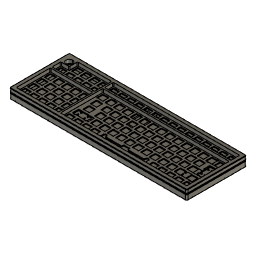
Varanidae (Autodesk Fusion 360 design; units mm, degrees)
Autodesk Fusion 360 part; units mm, degrees
(part 1 of 5)
sketch "スケッチ1" plane through (0, 0, 0) normal (0, 0, 1) x (1, 0, 0) in component "CasePlateDefault"
  spline S0 degree 3 poles (190.3558, 19.6941) (190.3558, 19.419) (190.1308, 19.194) (189.8555, 19.194) knots 0 0 0 0 1 1 1 1
  line L0 (189.8555, 19.194) -> (176.8555, 19.194)
  spline S1 degree 3 poles (176.8555, 19.194) (176.5806, 19.194) (176.3556, 19.419) (176.3556, 19.6941) knots 2 2 2 2 3 3 3 3
  line L1 (176.3556, 19.6941) -> (176.3556, 32.6938)
  spline S2 degree 3 poles (176.3556, 32.6938) (176.3556, 32.9689) (176.5806, 33.1939) (176.8555, 33.1939) knots 4 4 4 4 5 5 5 5
  line L2 (176.8555, 33.1939) -> (189.8555, 33.1939)
  spline S3 degree 3 poles (189.8555, 33.1939) (190.1308, 33.1939) (190.3558, 32.9689) (190.3558, 32.6938) knots 6 6 6 6 7 7 7 7
  line L3 (190.3558, 32.6938) -> (190.3558, 19.6941)
  spline S4 degree 3 poles (148.2805, 0.144) (148.0055, 0.144) (147.7806, 0.369) (147.7806, 0.6441) knots 0 0 0 0 1 1 1 1
  line L4 (147.7806, 0.6441) -> (147.7806, 13.6438)
  spline S5 degree 3 poles (147.7806, 13.6438) (147.7806, 13.9189) (148.0055, 14.1438) (148.2805, 14.1438) knots 2 2 2 2 3 3 3 3
  line L5 (148.2805, 14.1438) -> (161.2805, 14.1438)
  spline S6 degree 3 poles (161.2805, 14.1438) (161.5558, 14.1438) (161.7808, 13.9189) (161.7808, 13.6438) knots 4 4 4 4 5 5 5 5
  line L6 (161.7808, 13.6438) -> (161.7808, 0.6441)
  spline S7 degree 3 poles (161.7808, 0.6441) (161.7808, 0.369) (161.5558, 0.144) (161.2805, 0.144) knots 6 6 6 6 7 7 7 7
  line L7 (161.2805, 0.144) -> (148.2805, 0.144)
  spline S8 degree 3 poles (137.9686, -37.456) (137.9686, -37.7311) (137.7436, -37.956) (137.4684, -37.956) knots 0 0 0 0 1 1 1 1
  line L8 (137.4684, -37.956) -> (124.4686, -37.956)
  spline S9 degree 3 poles (124.4686, -37.956) (124.1937, -37.956) (123.9687, -37.7311) (123.9687, -37.456) knots 2 2 2 2 3 3 3 3
  line L9 (123.9687, -37.456) -> (123.9687, -24.4562)
  spline S10 degree 3 poles (123.9687, -24.4562) (123.9687, -24.1811) (124.1937, -23.9562) (124.4686, -23.9562) knots 4 4 4 4 5 5 5 5
  line L10 (124.4686, -23.9562) -> (137.4684, -23.9562)
  spline S11 degree 3 poles (137.4684, -23.9562) (137.7436, -23.9562) (137.9686, -24.1811) (137.9686, -24.4562) knots 6 6 6 6 7 7 7 7
  line L11 (137.9686, -24.4562) -> (137.9686, -37.456)
  spline S12 degree 3 poles (118.9186, -37.456) (118.9186, -37.7311) (118.6936, -37.956) (118.4183, -37.956) knots 0 0 0 0 1 1 1 1
  line L12 (118.4183, -37.956) -> (105.4186, -37.956)
  spline S13 degree 3 poles (105.4186, -37.956) (105.1437, -37.956) (104.9187, -37.7311) (104.9187, -37.456) knots 2 2 2 2 3 3 3 3
  line L13 (104.9187, -37.456) -> (104.9187, -24.4562)
  spline S14 degree 3 poles (104.9187, -24.4562) (104.9187, -24.1811) (105.1437, -23.9562) (105.4186, -23.9562) knots 4 4 4 4 5 5 5 5
  line L14 (105.4186, -23.9562) -> (118.4183, -23.9562)
  spline S15 degree 3 poles (118.4183, -23.9562) (118.6936, -23.9562) (118.9186, -24.1811) (118.9186, -24.4562) knots 6 6 6 6 7 7 7 7
  line L15 (118.9186, -24.4562) -> (118.9186, -37.456)
  spline S16 degree 3 poles (133.2057, -56.506) (133.2057, -56.7811) (132.9808, -57.006) (132.7055, -57.006) knots 0 0 0 0 1 1 1 1
  line L16 (132.7055, -57.006) -> (119.7054, -57.006)
  spline S17 degree 3 poles (119.7054, -57.006) (119.4305, -57.006) (119.2056, -56.7811) (119.2056, -56.506) knots 2 2 2 2 3 3 3 3
  line L17 (119.2056, -56.506) -> (119.2056, -43.5062)
  spline S18 degree 3 poles (119.2056, -43.5062) (119.2056, -43.2312) (119.4305, -43.0062) (119.7054, -43.0062) knots 4 4 4 4 5 5 5 5
  line L18 (119.7054, -43.0062) -> (132.7055, -43.0062)
  spline S19 degree 3 poles (132.7055, -43.0062) (132.9808, -43.0062) (133.2057, -43.2312) (133.2057, -43.5062) knots 6 6 6 6 7 7 7 7
  line L19 (133.2057, -43.5062) -> (133.2057, -56.506)
  line L20 (198.3818, 67.532) -> (-198.3818, 67.532)
  spline S20 degree 3 poles (-198.3818, 67.532) (-199.7568, 67.532) (-200.8816, 66.407) (-200.8816, 65.0321) knots 1 1 1 1 2 2 2 2
  line L21 (-200.8816, 65.0321) -> (-200.8816, -65.0319)
  spline S21 degree 3 poles (-200.8816, -65.0319) (-200.8816, -66.4072) (-199.7568, -67.532) (-198.3818, -67.532) knots 3 3 3 3 4 4 4 4
  line L22 (-198.3818, -67.532) -> (198.3818, -67.532)
  spline S22 degree 3 poles (198.3818, -67.532) (199.7564, -67.532) (200.8816, -66.4072) (200.8816, -65.0319) knots 5 5 5 5 6 6 6 6
  line L23 (200.8816, -65.0319) -> (200.8816, 65.0321)
  spline S23 degree 3 poles (200.8816, 65.0321) (200.8816, 66.407) (199.7564, 67.532) (198.3818, 67.532) knots 7 7 7 7 8 8 8 8
  spline S24 degree 3 poles (171.3058, -56.506) (171.3058, -56.7811) (171.0808, -57.006) (170.8055, -57.006) knots 0 0 0 0 1 1 1 1
  line L24 (170.8055, -57.006) -> (157.8055, -57.006)
  spline S25 degree 3 poles (157.8055, -57.006) (157.5305, -57.006) (157.3056, -56.7811) (157.3056, -56.506) knots 2 2 2 2 3 3 3 3
  line L25 (157.3056, -56.506) -> (157.3056, -43.5062)
  spline S26 degree 3 poles (157.3056, -43.5062) (157.3056, -43.2312) (157.5305, -43.0062) (157.8055, -43.0062) knots 4 4 4 4 5 5 5 5
  line L26 (157.8055, -43.0062) -> (170.8055, -43.0062)
  spline S27 degree 3 poles (170.8055, -43.0062) (171.0808, -43.0062) (171.3058, -43.2312) (171.3058, -43.5062) knots 6 6 6 6 7 7 7 7
  line L27 (171.3058, -43.5062) -> (171.3058, -56.506)
  spline S28 degree 3 poles (190.3558, -56.506) (190.3558, -56.7811) (190.1308, -57.006) (189.8555, -57.006) knots 0 0 0 0 1 1 1 1
  line L28 (189.8555, -57.006) -> (176.8555, -57.006)
  spline S29 degree 3 poles (176.8555, -57.006) (176.5806, -57.006) (176.3556, -56.7811) (176.3556, -56.506) knots 2 2 2 2 3 3 3 3
  line L29 (176.3556, -56.506) -> (176.3556, -43.5062)
  spline S30 degree 3 poles (176.3556, -43.5062) (176.3556, -43.2312) (176.5806, -43.0062) (176.8555, -43.0062) knots 4 4 4 4 5 5 5 5
  line L30 (176.8555, -43.0062) -> (189.8555, -43.0062)
  spline S31 degree 3 poles (189.8555, -43.0062) (190.1308, -43.0062) (190.3558, -43.2312) (190.3558, -43.5062) knots 6 6 6 6 7 7 7 7
  line L31 (190.3558, -43.5062) -> (190.3558, -56.506)
  spline S32 degree 3 poles (157.3056, 56.506) (157.3056, 56.7811) (157.5305, 57.006) (157.8055, 57.006) knots 0 0 0 0 1 1 1 1
  line L32 (157.8055, 57.006) -> (170.8055, 57.006)
  spline S33 degree 3 poles (170.8055, 57.006) (171.0808, 57.006) (171.3058, 56.7811) (171.3058, 56.506) knots 2 2 2 2 3 3 3 3
  line L33 (171.3058, 56.506) -> (171.3058, 43.5059)
  spline S34 degree 3 poles (171.3058, 43.5059) (171.3058, 43.2308) (171.0808, 43.0058) (170.8055, 43.0058) knots 4 4 4 4 5 5 5 5
  line L34 (170.8055, 43.0058) -> (157.8055, 43.0058)
  spline S35 degree 3 poles (157.8055, 43.0058) (157.5305, 43.0058) (157.3056, 43.2308) (157.3056, 43.5059) knots 6 6 6 6 7 7 7 7
  line L35 (157.3056, 43.5059) -> (157.3056, 56.506)
  spline S36 degree 3 poles (157.3056, 32.6938) (157.3056, 32.9689) (157.5305, 33.1939) (157.8055, 33.1939) knots 0 0 0 0 1 1 1 1
  line L36 (157.8055, 33.1939) -> (170.8055, 33.1939)
  spline S37 degree 3 poles (170.8055, 33.1939) (171.0808, 33.1939) (171.3058, 32.9689) (171.3058, 32.6938) knots 2 2 2 2 3 3 3 3
  line L37 (171.3058, 32.6938) -> (171.3058, 19.6941)
  spline S38 degree 3 poles (171.3058, 19.6941) (171.3058, 19.419) (171.0808, 19.194) (170.8055, 19.194) knots 4 4 4 4 5 5 5 5
  line L38 (170.8055, 19.194) -> (157.8055, 19.194)
  spline S39 degree 3 poles (157.8055, 19.194) (157.5305, 19.194) (157.3056, 19.419) (157.3056, 19.6941) knots 6 6 6 6 7 7 7 7
  line L39 (157.3056, 19.6941) -> (157.3056, 32.6938)
  spline S40 degree 3 poles (157.0186, -37.456) (157.0186, -37.7311) (156.7936, -37.956) (156.5184, -37.956) knots 0 0 0 0 1 1 1 1
  line L40 (156.5184, -37.956) -> (143.5186, -37.956)
  spline S41 degree 3 poles (143.5186, -37.956) (143.2437, -37.956) (143.0188, -37.7311) (143.0188, -37.456) knots 2 2 2 2 3 3 3 3
  line L41 (143.0188, -37.456) -> (143.0188, -24.4562)
  spline S42 degree 3 poles (143.0188, -24.4562) (143.0188, -24.1811) (143.2437, -23.9562) (143.5186, -23.9562) knots 4 4 4 4 5 5 5 5
  line L42 (143.5186, -23.9562) -> (156.5184, -23.9562)
  spline S43 degree 3 poles (156.5184, -23.9562) (156.7936, -23.9562) (157.0186, -24.1811) (157.0186, -24.4562) knots 6 6 6 6 7 7 7 7
  line L43 (157.0186, -24.4562) -> (157.0186, -37.456)
  line L44 (183.2117, -24.4562) -> (183.2117, -37.456)
  spline S44 degree 3 poles (183.2117, -37.456) (183.2117, -37.7311) (182.9867, -37.956) (182.7114, -37.956) knots 1 1 1 1 2 2 2 2
  line L45 (182.7114, -37.956) -> (169.7114, -37.956)
  spline S45 degree 3 poles (169.7114, -37.956) (169.4365, -37.956) (169.2115, -37.7311) (169.2115, -37.456) knots 3 3 3 3 4 4 4 4
  line L46 (169.2115, -37.456) -> (169.2115, -24.4562)
  spline S46 degree 3 poles (169.2115, -24.4562) (169.2115, -24.1811) (169.4365, -23.9562) (169.7114, -23.9562) knots 5 5 5 5 6 6 6 6
  line L47 (169.7114, -23.9562) -> (182.7114, -23.9562)
  spline S47 degree 3 poles (182.7114, -23.9562) (182.9867, -23.9562) (183.2117, -24.1811) (183.2117, -24.4562) knots 7 7 7 7 8 8 8 8
  spline S48 degree 3 poles (190.3558, 43.5059) (190.3558, 43.2308) (190.1308, 43.0058) (189.8555, 43.0058) knots 0 0 0 0 1 1 1 1
  line L48 (189.8555, 43.0058) -> (176.8555, 43.0058)
  spline S49 degree 3 poles (176.8555, 43.0058) (176.5806, 43.0058) (176.3556, 43.2308) (176.3556, 43.5059) knots 2 2 2 2 3 3 3 3
  line L49 (176.3556, 43.5059) -> (176.3556, 56.506)
  spline S50 degree 3 poles (176.3556, 56.506) (176.3556, 56.7811) (176.5806, 57.006) (176.8555, 57.006) knots 4 4 4 4 5 5 5 5
  line L50 (176.8555, 57.006) -> (189.8555, 57.006)
  spline S51 degree 3 poles (189.8555, 57.006) (190.1308, 57.006) (190.3558, 56.7811) (190.3558, 56.506) knots 6 6 6 6 7 7 7 7
  line L51 (190.3558, 56.506) -> (190.3558, 43.5059)
  spline S52 degree 3 poles (152.2558, -56.506) (152.2558, -56.7811) (152.0308, -57.006) (151.7555, -57.006) knots 0 0 0 0 1 1 1 1
  line L52 (151.7555, -57.006) -> (138.7554, -57.006)
  spline S53 degree 3 poles (138.7554, -57.006) (138.4805, -57.006) (138.2556, -56.7811) (138.2556, -56.506) knots 2 2 2 2 3 3 3 3
  line L53 (138.2556, -56.506) -> (138.2556, -43.5062)
  spline S54 degree 3 poles (138.2556, -43.5062) (138.2556, -43.2312) (138.4805, -43.0062) (138.7554, -43.0062) knots 4 4 4 4 5 5 5 5
  line L54 (138.7554, -43.0062) -> (151.7555, -43.0062)
  spline S55 degree 3 poles (151.7555, -43.0062) (152.0308, -43.0062) (152.2558, -43.2312) (152.2558, -43.5062) knots 6 6 6 6 7 7 7 7
  line L55 (152.2558, -43.5062) -> (152.2558, -56.506)
  spline S56 degree 3 poles (173.0045, -13.0311) (173.0045, -12.756) (173.2295, -12.531) (173.5044, -12.531) knots 0 0 0 0 1 1 1 1
  line L56 (173.5044, -12.531) -> (173.7042, -12.531)
  spline S57 degree 3 poles (173.7042, -12.531) (173.9795, -12.531) (174.2045, -12.3061) (174.2045, -12.031) knots 2 2 2 2 3 3 3 3
  line L57 (174.2045, -12.031) -> (174.2045, -11.3061)
  spline S58 degree 3 poles (174.2045, -11.3061) (174.2045, -11.031) (174.4294, -10.8061) (174.7044, -10.8061) knots 4 4 4 4 5 5 5 5
  line L58 (174.7044, -10.8061) -> (178.1746, -10.8061)
  spline S59 degree 3 poles (178.1746, -10.8061) (178.4499, -10.8061) (178.6748, -10.5811) (178.6748, -10.306) knots 6 6 6 6 7 7 7 7
  line L59 (178.6748, -10.306) -> (178.6748, -9.8811)
  spline S60 degree 3 poles (178.6748, -9.8811) (178.6748, -9.606) (178.4499, -9.381) (178.1746, -9.381) knots 8 8 8 8 9 9 9 9
  line L60 (178.1746, -9.381) -> (174.4746, -9.381)
  spline S61 degree 3 poles (174.4746, -9.381) (174.1996, -9.381) (173.9747, -9.156) (173.9747, -8.8809) knots 10 10 10 10 11 11 11 11
  line L61 (173.9747, -8.8809) -> (173.9747, 4.1188)
  spline S62 degree 3 poles (173.9747, 4.1188) (173.9747, 4.3939) (174.1996, 4.6188) (174.4746, 4.6188) knots 12 12 12 12 13 13 13 13
  line L62 (174.4746, 4.6188) -> (178.1746, 4.6188)
  spline S63 degree 3 poles (178.1746, 4.6188) (178.4499, 4.6188) (178.6748, 4.8438) (178.6748, 5.1189) knots 14 14 14 14 15 15 15 15
  line L63 (178.6748, 5.1189) -> (178.6748, 5.544)
  spline S64 degree 3 poles (178.6748, 5.544) (178.6748, 5.8191) (178.4499, 6.0441) (178.1746, 6.0441) knots 16 16 16 16 17 17 17 17
  line L64 (178.1746, 6.0441) -> (174.7044, 6.0441)
  spline S65 degree 3 poles (174.7044, 6.0441) (174.4294, 6.0441) (174.2045, 6.269) (174.2045, 6.5441) knots 18 18 18 18 19 19 19 19
  line L65 (174.2045, 6.5441) -> (174.2045, 7.269)
  spline S66 degree 3 poles (174.2045, 7.269) (174.2045, 7.5441) (173.9795, 7.769) (173.7042, 7.769) knots 20 20 20 20 21 21 21 21
  line L66 (173.7042, 7.769) -> (173.5044, 7.769)
  spline S67 degree 3 poles (173.5044, 7.769) (173.2295, 7.769) (173.0045, 7.994) (173.0045, 8.2691) knots 22 22 22 22 23 23 23 23
  line L67 (173.0045, 8.2691) -> (173.0045, 10.9189)
  spline S68 degree 3 poles (173.0045, 10.9189) (173.0045, 11.194) (173.2295, 11.4189) (173.5044, 11.4189) knots 24 24 24 24 25 25 25 25
  line L68 (173.5044, 11.4189) -> (173.7042, 11.4189)
  spline S69 degree 3 poles (173.7042, 11.4189) (173.9795, 11.4189) (174.2045, 11.6439) (174.2045, 11.919) knots 26 26 26 26 27 27 27 27
  line L69 (174.2045, 11.919) -> (174.2045, 12.644)
  spline S70 degree 3 poles (174.2045, 12.644) (174.2045, 12.9191) (174.4294, 13.1441) (174.7044, 13.1441) knots 28 28 28 28 29 29 29 29
  line L70 (174.7044, 13.1441) -> (179.9743, 13.1441)
  spline S71 degree 3 poles (179.9743, 13.1441) (180.2496, 13.1441) (180.4745, 13.2734) (180.4745, 13.5897) (180.6995, 13.7191) (180.9744, 13.7191) knots 30 30 30 30 31 31 32 32 32 32
  line L71 (180.9744, 13.7191) -> (182.7745, 13.7191)
  spline S72 degree 3 poles (182.7745, 13.7191) (183.0498, 13.7191) (183.2747, 13.5897) (183.2747, 13.2734) (183.4997, 13.1441) (183.7746, 13.1441) knots 33 33 33 33 34 34 35 35 35 35
  line L72 (183.7746, 13.1441) -> (186.5038, 13.1441)
  spline S73 degree 3 poles (186.5038, 13.1441) (186.7791, 13.1441) (187.004, 12.9191) (187.004, 12.644) knots 36 36 36 36 37 37 37 37
  line L73 (187.004, 12.644) -> (187.004, 6.5441)
  spline S74 degree 3 poles (187.004, 6.5441) (187.004, 6.269) (186.7791, 6.0441) (186.5038, 6.0441) knots 38 38 38 38 39 39 39 39
  line L74 (186.5038, 6.0441) -> (183.7746, 6.0441)
  spline S75 degree 3 poles (183.7746, 6.0441) (183.4997, 6.0441) (183.2747, 5.8191) (183.2747, 5.544) knots 40 40 40 40 41 41 41 41
  line L75 (183.2747, 5.544) -> (183.2747, 5.1189)
  spline S76 degree 3 poles (183.2747, 5.1189) (183.2747, 4.8438) (183.4997, 4.6188) (183.7746, 4.6188) knots 42 42 42 42 43 43 43 43
  line L76 (183.7746, 4.6188) -> (187.4743, 4.6188)
  spline S77 degree 3 poles (187.4743, 4.6188) (187.7496, 4.6188) (187.9745, 4.3939) (187.9745, 4.1188) knots 44 44 44 44 45 45 45 45
  line L77 (187.9745, 4.1188) -> (187.9745, -8.8809)
  spline S78 degree 3 poles (187.9745, -8.8809) (187.9745, -9.156) (187.7496, -9.381) (187.4743, -9.381) knots 46 46 46 46 47 47 47 47
  line L78 (187.4743, -9.381) -> (183.7746, -9.381)
  spline S79 degree 3 poles (183.7746, -9.381) (183.4997, -9.381) (183.2747, -9.606) (183.2747, -9.8811) knots 48 48 48 48 49 49 49 49
  line L79 (183.2747, -9.8811) -> (183.2747, -10.306)
  spline S80 degree 3 poles (183.2747, -10.306) (183.2747, -10.5811) (183.4997, -10.8061) (183.7746, -10.8061) knots 50 50 50 50 51 51 51 51
  line L80 (183.7746, -10.8061) -> (186.5038, -10.8061)
  spline S81 degree 3 poles (186.5038, -10.8061) (186.7791, -10.8061) (187.004, -11.031) (187.004, -11.3061) knots 52 52 52 52 53 53 53 53
  line L81 (187.004, -11.3061) -> (187.004, -17.406)
  spline S82 degree 3 poles (187.004, -17.406) (187.004, -17.6811) (186.7791, -17.9061) (186.5038, -17.9061) knots 54 54 54 54 55 55 55 55
  line L82 (186.5038, -17.9061) -> (183.7746, -17.9061)
  spline S83 degree 3 poles (183.7746, -17.9061) (183.4997, -17.9061) (183.2747, -18.0354) (183.2747, -18.1936) (183.2747, -18.3519) (183.0498, -18.4812) (182.7745, -18.4812) knots 56 56 56 56 57 57 57 58 58 58 58
  line L83 (182.7745, -18.4812) -> (180.9744, -18.4812)
  spline S84 degree 3 poles (180.9744, -18.4812) (180.6995, -18.4812) (180.4745, -18.3519) (180.4745, -18.1936) (180.4745, -18.0354) (180.2496, -17.9061) (179.9743, -17.9061) knots 59 59 59 59 60 60 60 61 61 61 61
  line L84 (179.9743, -17.9061) -> (174.7044, -17.9061)
  spline S85 degree 3 poles (174.7044, -17.9061) (174.4294, -17.9061) (174.2045, -17.6811) (174.2045, -17.406) knots 62 62 62 62 63 63 63 63
  line L85 (174.2045, -17.406) -> (174.2045, -16.681)
  spline S86 degree 3 poles (174.2045, -16.681) (174.2045, -16.4059) (173.9795, -16.1809) (173.7042, -16.1809) knots 64 64 64 64 65 65 65 65
  line L86 (173.7042, -16.1809) -> (173.5044, -16.1809)
  spline S87 degree 3 poles (173.5044, -16.1809) (173.2295, -16.1809) (173.0045, -15.956) (173.0045, -15.6809) knots 66 66 66 66 67 67 67 67
  line L87 (173.0045, -15.6809) -> (173.0045, -13.0311)
  spline S88 degree 3 poles (152.5438, -5.4062) (152.5438, -5.1311) (152.7687, -4.9062) (153.0436, -4.9062) knots 0 0 0 0 1 1 1 1
  line L88 (153.0436, -4.9062) -> (166.0434, -4.9062)
  spline S89 degree 3 poles (166.0434, -4.9062) (166.3186, -4.9062) (166.5436, -5.1311) (166.5436, -5.4062) knots 2 2 2 2 3 3 3 3
  line L89 (166.5436, -5.4062) -> (166.5436, -18.406)
  spline S90 degree 3 poles (166.5436, -18.406) (166.5436, -18.681) (166.3186, -18.906) (166.0434, -18.906) knots 4 4 4 4 5 5 5 5
  line L90 (166.0434, -18.906) -> (153.0436, -18.906)
  spline S91 degree 3 poles (153.0436, -18.906) (152.7687, -18.906) (152.5438, -18.681) (152.5438, -18.406) knots 6 6 6 6 7 7 7 7
  line L91 (152.5438, -18.406) -> (152.5438, -5.4062)
  spline S92 degree 3 poles (138.2556, 32.6938) (138.2556, 32.9689) (138.4805, 33.1939) (138.7554, 33.1939) knots 0 0 0 0 1 1 1 1
  line L92 (138.7554, 33.1939) -> (151.7555, 33.1939)
  spline S93 degree 3 poles (151.7555, 33.1939) (152.0308, 33.1939) (152.2558, 32.9689) (152.2558, 32.6938) knots 2 2 2 2 3 3 3 3
  line L93 (152.2558, 32.6938) -> (152.2558, 19.6941)
  spline S94 degree 3 poles (152.2558, 19.6941) (152.2558, 19.419) (152.0308, 19.194) (151.7555, 19.194) knots 4 4 4 4 5 5 5 5
  line L94 (151.7555, 19.194) -> (138.7554, 19.194)
  spline S95 degree 3 poles (138.7554, 19.194) (138.4805, 19.194) (138.2556, 19.419) (138.2556, 19.6941) knots 6 6 6 6 7 7 7 7
  line L95 (138.2556, 19.6941) -> (138.2556, 32.6938)
  spline S96 degree 3 poles (138.2556, 56.506) (138.2556, 56.7811) (138.4805, 57.006) (138.7554, 57.006) knots 0 0 0 0 1 1 1 1
  line L96 (138.7554, 57.006) -> (151.7555, 57.006)
  spline S97 degree 3 poles (151.7555, 57.006) (152.0308, 57.006) (152.2558, 56.7811) (152.2558, 56.506) knots 2 2 2 2 3 3 3 3
  line L97 (152.2558, 56.506) -> (152.2558, 43.5059)
  spline S98 degree 3 poles (152.2558, 43.5059) (152.2558, 43.2308) (152.0308, 43.0058) (151.7555, 43.0058) knots 4 4 4 4 5 5 5 5
  line L98 (151.7555, 43.0058) -> (138.7554, 43.0058)
  spline S99 degree 3 poles (138.7554, 43.0058) (138.4805, 43.0058) (138.2556, 43.2308) (138.2556, 43.5059) knots 6 6 6 6 7 7 7 7
  line L99 (138.2556, 43.5059) -> (138.2556, 56.506)
  spline S100 degree 3 poles (-71.2946, 32.6938) (-71.2946, 32.9689) (-71.0696, 33.1939) (-70.7947, 33.1939) knots 0 0 0 0 1 1 1 1
  line L100 (-70.7947, 33.1939) -> (-57.795, 33.1939)
  spline S101 degree 3 poles (-57.795, 33.1939) (-57.5197, 33.1939) (-57.2947, 32.9689) (-57.2947, 32.6938) knots 2 2 2 2 3 3 3 3
  line L101 (-57.2947, 32.6938) -> (-57.2947, 19.6941)
  spline S102 degree 3 poles (-57.2947, 19.6941) (-57.2947, 19.419) (-57.5197, 19.194) (-57.795, 19.194) knots 4 4 4 4 5 5 5 5
  line L102 (-57.795, 19.194) -> (-70.7947, 19.194)
  spline S103 degree 3 poles (-70.7947, 19.194) (-71.0696, 19.194) (-71.2946, 19.419) (-71.2946, 19.6941) knots 6 6 6 6 7 7 7 7
  line L103 (-71.2946, 19.6941) -> (-71.2946, 32.6938)
  spline S104 degree 3 poles (-71.2946, 56.506) (-71.2946, 56.7811) (-71.0696, 57.006) (-70.7947, 57.006) knots 0 0 0 0 1 1 1 1
  line L104 (-70.7947, 57.006) -> (-57.795, 57.006)
  spline S105 degree 3 poles (-57.795, 57.006) (-57.5197, 57.006) (-57.2947, 56.7811) (-57.2947, 56.506) knots 2 2 2 2 3 3 3 3
  line L105 (-57.2947, 56.506) -> (-57.2947, 43.5059)
  spline S106 degree 3 poles (-57.2947, 43.5059) (-57.2947, 43.2308) (-57.5197, 43.0058) (-57.795, 43.0058) knots 4 4 4 4 5 5 5 5
  line L106 (-57.795, 43.0058) -> (-70.7947, 43.0058)
  spline S107 degree 3 poles (-70.7947, 43.0058) (-71.0696, 43.0058) (-71.2946, 43.2308) (-71.2946, 43.5059) knots 6 6 6 6 7 7 7 7
  line L107 (-71.2946, 43.5059) -> (-71.2946, 56.506)
  line L108 (-69.2006, -5.4062) -> (-69.2006, -18.406)
  spline S108 degree 3 poles (-69.2006, -18.406) (-69.2006, -18.681) (-69.4256, -18.906) (-69.7009, -18.906) knots 1 1 1 1 2 2 2 2
  line L109 (-69.7009, -18.906) -> (-82.7006, -18.906)
  spline S109 degree 3 poles (-82.7006, -18.906) (-82.9755, -18.906) (-83.2005, -18.681) (-83.2005, -18.406) knots 3 3 3 3 4 4 4 4
  line L110 (-83.2005, -18.406) -> (-83.2005, -5.4062)
  spline S110 degree 3 poles (-83.2005, -5.4062) (-83.2005, -5.1311) (-82.9755, -4.9062) (-82.7006, -4.9062) knots 5 5 5 5 6 6 6 6
  line L111 (-82.7006, -4.9062) -> (-69.7009, -4.9062)
  spline S111 degree 3 poles (-69.7009, -4.9062) (-69.4256, -4.9062) (-69.2006, -5.1311) (-69.2006, -5.4062) knots 7 7 7 7 8 8 8 8
  line L112 (14.4305, 0.6441) -> (14.4305, 13.6438)
  spline S112 degree 3 poles (14.4305, 13.6438) (14.4305, 13.9189) (14.6554, 14.1438) (14.9304, 14.1438) knots 1 1 1 1 2 2 2 2
  line L113 (14.9304, 14.1438) -> (27.9304, 14.1438)
  spline S113 degree 3 poles (27.9304, 14.1438) (28.2057, 14.1438) (28.4307, 13.9189) (28.4307, 13.6438) knots 3 3 3 3 4 4 4 4
  line L114 (28.4307, 13.6438) -> (28.4307, 0.6441)
  spline S114 degree 3 poles (28.4307, 0.6441) (28.4307, 0.369) (28.2057, 0.144) (27.9304, 0.144) knots 5 5 5 5 6 6 6 6
  line L115 (27.9304, 0.144) -> (14.9304, 0.144)
  spline S115 degree 3 poles (14.9304, 0.144) (14.6554, 0.144) (14.4305, 0.369) (14.4305, 0.6441) knots 7 7 7 7 8 8 8 8
  spline S116 degree 3 poles (133.4937, -5.4062) (133.4937, -5.1311) (133.7187, -4.9062) (133.9936, -4.9062) knots 0 0 0 0 1 1 1 1
  line L116 (133.9936, -4.9062) -> (146.9934, -4.9062)
  spline S117 degree 3 poles (146.9934, -4.9062) (147.2686, -4.9062) (147.4936, -5.1311) (147.4936, -5.4062) knots 2 2 2 2 3 3 3 3
  line L117 (147.4936, -5.4062) -> (147.4936, -18.406)
  spline S118 degree 3 poles (147.4936, -18.406) (147.4936, -18.681) (147.2686, -18.906) (146.9934, -18.906) knots 4 4 4 4 5 5 5 5
  line L118 (146.9934, -18.906) -> (133.9936, -18.906)
  spline S119 degree 3 poles (133.9936, -18.906) (133.7187, -18.906) (133.4937, -18.681) (133.4937, -18.406) knots 6 6 6 6 7 7 7 7
  line L119 (133.4937, -18.406) -> (133.4937, -5.4062)
  line L120 (-71.5816, 13.6438) -> (-71.5816, 0.6441)
  spline S120 degree 3 poles (-71.5816, 0.6441) (-71.5816, 0.369) (-71.8065, 0.144) (-72.0818, 0.144) knots 1 1 1 1 2 2 2 2
  line L121 (-72.0818, 0.144) -> (-85.0819, 0.144)
  spline S121 degree 3 poles (-85.0819, 0.144) (-85.3568, 0.144) (-85.5817, 0.369) (-85.5817, 0.6441) knots 3 3 3 3 4 4 4 4
  line L122 (-85.5817, 0.6441) -> (-85.5817, 13.6438)
  spline S122 degree 3 poles (-85.5817, 13.6438) (-85.5817, 13.9189) (-85.3568, 14.1438) (-85.0819, 14.1438) knots 5 5 5 5 6 6 6 6
  line L123 (-85.0819, 14.1438) -> (-72.0818, 14.1438)
  spline S123 degree 3 poles (-72.0818, 14.1438) (-71.8065, 14.1438) (-71.5816, 13.9189) (-71.5816, 13.6438) knots 7 7 7 7 8 8 8 8
  spline S124 degree 3 poles (47.7687, -24.4562) (47.7687, -24.1811) (47.9937, -23.9562) (48.2686, -23.9562) knots 0 0 0 0 1 1 1 1
  line L124 (48.2686, -23.9562) -> (61.2673, -23.9562)
  spline S125 degree 3 poles (61.2673, -23.9562) (61.5425, -23.9562) (61.7675, -24.1811) (61.7675, -24.4562) knots 2 2 2 2 3 3 3 3
  line L125 (61.7675, -24.4562) -> (61.7675, -37.456)
  spline S126 degree 3 poles (61.7675, -37.456) (61.7675, -37.7311) (61.5425, -37.956) (61.2673, -37.956) knots 4 4 4 4 5 5 5 5
  line L126 (61.2673, -37.956) -> (48.2686, -37.956)
  spline S127 degree 3 poles (48.2686, -37.956) (47.9937, -37.956) (47.7687, -37.7311) (47.7687, -37.456) knots 6 6 6 6 7 7 7 7
  line L127 (47.7687, -37.456) -> (47.7687, -24.4562)
  spline S128 degree 3 poles (-90.3446, 56.506) (-90.3446, 56.7811) (-90.1196, 57.006) (-89.8447, 57.006) knots 0 0 0 0 1 1 1 1
  line L128 (-89.8447, 57.006) -> (-76.845, 57.006)
  spline S129 degree 3 poles (-76.845, 57.006) (-76.5697, 57.006) (-76.3447, 56.7811) (-76.3447, 56.506) knots 2 2 2 2 3 3 3 3
  line L129 (-76.3447, 56.506) -> (-76.3447, 43.5059)
  spline S130 degree 3 poles (-76.3447, 43.5059) (-76.3447, 43.2308) (-76.5697, 43.0058) (-76.845, 43.0058) knots 4 4 4 4 5 5 5 5
  line L130 (-76.845, 43.0058) -> (-89.8447, 43.0058)
  spline S131 degree 3 poles (-89.8447, 43.0058) (-90.1196, 43.0058) (-90.3446, 43.2308) (-90.3446, 43.5059) knots 6 6 6 6 7 7 7 7
  line L131 (-90.3446, 43.5059) -> (-90.3446, 56.506)
  spline S132 degree 3 poles (119.2056, 56.506) (119.2056, 56.7811) (119.4305, 57.006) (119.7054, 57.006) knots 0 0 0 0 1 1 1 1
  line L132 (119.7054, 57.006) -> (132.7055, 57.006)
  spline S133 degree 3 poles (132.7055, 57.006) (132.9808, 57.006) (133.2057, 56.7811) (133.2057, 56.506) knots 2 2 2 2 3 3 3 3
  line L133 (133.2057, 56.506) -> (133.2057, 43.5059)
  spline S134 degree 3 poles (133.2057, 43.5059) (133.2057, 43.2308) (132.9808, 43.0058) (132.7055, 43.0058) knots 4 4 4 4 5 5 5 5
  line L134 (132.7055, 43.0058) -> (119.7054, 43.0058)
  spline S135 degree 3 poles (119.7054, 43.0058) (119.4305, 43.0058) (119.2056, 43.2308) (119.2056, 43.5059) knots 6 6 6 6 7 7 7 7
  line L135 (119.2056, 43.5059) -> (119.2056, 56.506)
  spline S136 degree 3 poles (-18.9064, -5.4062) (-18.9064, -5.1311) (-18.6814, -4.9062) (-18.4065, -4.9062) knots 0 0 0 0 1 1 1 1
  line L136 (-18.4065, -4.9062) -> (-5.4067, -4.9062)
  spline S137 degree 3 poles (-5.4067, -4.9062) (-5.1315, -4.9062) (-4.9065, -5.1311) (-4.9065, -5.4062) knots 2 2 2 2 3 3 3 3
  line L137 (-4.9065, -5.4062) -> (-4.9065, -18.406)
  spline S138 degree 3 poles (-4.9065, -18.406) (-4.9065, -18.681) (-5.1315, -18.906) (-5.4067, -18.906) knots 4 4 4 4 5 5 5 5
  line L138 (-5.4067, -18.906) -> (-18.4065, -18.906)
  spline S139 degree 3 poles (-18.4065, -18.906) (-18.6814, -18.906) (-18.9064, -18.681) (-18.9064, -18.406) knots 6 6 6 6 7 7 7 7
  line L139 (-18.9064, -18.406) -> (-18.9064, -5.4062)
  spline S140 degree 3 poles (28.7187, -24.4562) (28.7187, -24.1811) (28.9436, -23.9562) (29.2186, -23.9562) knots 0 0 0 0 1 1 1 1
  line L140 (29.2186, -23.9562) -> (42.2183, -23.9562)
  spline S141 degree 3 poles (42.2183, -23.9562) (42.4936, -23.9562) (42.7185, -24.1811) (42.7185, -24.4562) knots 2 2 2 2 3 3 3 3
  line L141 (42.7185, -24.4562) -> (42.7185, -37.456)
  spline S142 degree 3 poles (42.7185, -37.456) (42.7185, -37.7311) (42.4936, -37.956) (42.2183, -37.956) knots 4 4 4 4 5 5 5 5
  line L142 (42.2183, -37.956) -> (29.2186, -37.956)
  spline S143 degree 3 poles (29.2186, -37.956) (28.9436, -37.956) (28.7187, -37.7311) (28.7187, -37.456) knots 6 6 6 6 7 7 7 7
  line L143 (28.7187, -37.456) -> (28.7187, -24.4562)
  spline S144 degree 3 poles (-176.3566, -56.506) (-176.3566, -56.7811) (-176.5816, -57.006) (-176.8568, -57.006) knots 0 0 0 0 1 1 1 1
  line L144 (-176.8568, -57.006) -> (-189.8569, -57.006)
  spline S145 degree 3 poles (-189.8569, -57.006) (-190.1318, -57.006) (-190.3568, -56.7811) (-190.3568, -56.506) knots 2 2 2 2 3 3 3 3
  line L145 (-190.3568, -56.506) -> (-190.3568, -43.5062)
  spline S146 degree 3 poles (-190.3568, -43.5062) (-190.3568, -43.2312) (-190.1318, -43.0062) (-189.8569, -43.0062) knots 4 4 4 4 5 5 5 5
  line L146 (-189.8569, -43.0062) -> (-176.8568, -43.0062)
  spline S147 degree 3 poles (-176.8568, -43.0062) (-176.5816, -43.0062) (-176.3566, -43.2312) (-176.3566, -43.5062) knots 6 6 6 6 7 7 7 7
  line L147 (-176.3566, -43.5062) -> (-176.3566, -56.506)
  line L148 (52.5305, 0.6441) -> (52.5305, 13.6438)
  spline S148 degree 3 poles (52.5305, 13.6438) (52.5305, 13.9189) (52.7555, 14.1438) (53.0304, 14.1438) knots 1 1 1 1 2 2 2 2
  line L149 (53.0304, 14.1438) -> (66.0305, 14.1438)
  spline S149 degree 3 poles (66.0305, 14.1438) (66.3057, 14.1438) (66.5307, 13.9189) (66.5307, 13.6438) knots 3 3 3 3 4 4 4 4
  line L150 (66.5307, 13.6438) -> (66.5307, 0.6441)
  spline S150 degree 3 poles (66.5307, 0.6441) (66.5307, 0.369) (66.3057, 0.144) (66.0305, 0.144) knots 5 5 5 5 6 6 6 6
  line L151 (66.0305, 0.144) -> (53.0304, 0.144)
  spline S151 degree 3 poles (53.0304, 0.144) (52.7555, 0.144) (52.5305, 0.369) (52.5305, 0.6441) knots 7 7 7 7 8 8 8 8
  line L152 (-4.6195, 0.6441) -> (-4.6195, 13.6438)
  spline S152 degree 3 poles (-4.6195, 13.6438) (-4.6195, 13.9189) (-4.3946, 14.1438) (-4.1196, 14.1438) knots 1 1 1 1 2 2 2 2
  line L153 (-4.1196, 14.1438) -> (8.8804, 14.1438)
  spline S153 degree 3 poles (8.8804, 14.1438) (9.1557, 14.1438) (9.3807, 13.9189) (9.3807, 13.6438) knots 3 3 3 3 4 4 4 4
  line L154 (9.3807, 13.6438) -> (9.3807, 0.6441)
  spline S154 degree 3 poles (9.3807, 0.6441) (9.3807, 0.369) (9.1557, 0.144) (8.8804, 0.144) knots 5 5 5 5 6 6 6 6
  line L155 (8.8804, 0.144) -> (-4.1196, 0.144)
  spline S155 degree 3 poles (-4.1196, 0.144) (-4.3946, 0.144) (-4.6195, 0.369) (-4.6195, 0.6441) knots 7 7 7 7 8 8 8 8
  spline S156 degree 3 poles (-176.3566, -37.456) (-176.3566, -37.7311) (-176.5816, -37.956) (-176.8568, -37.956) knots 0 0 0 0 1 1 1 1
  line L156 (-176.8568, -37.956) -> (-189.8569, -37.956)
  spline S157 degree 3 poles (-189.8569, -37.956) (-190.1318, -37.956) (-190.3568, -37.7311) (-190.3568, -37.456) knots 2 2 2 2 3 3 3 3
  line L157 (-190.3568, -37.456) -> (-190.3568, -24.4562)
  spline S158 degree 3 poles (-190.3568, -24.4562) (-190.3568, -24.1811) (-190.1318, -23.9562) (-189.8569, -23.9562) knots 4 4 4 4 5 5 5 5
  line L158 (-189.8569, -23.9562) -> (-176.8568, -23.9562)
  spline S159 degree 3 poles (-176.8568, -23.9562) (-176.5816, -23.9562) (-176.3566, -24.1811) (-176.3566, -24.4562) knots 6 6 6 6 7 7 7 7
  line L159 (-176.3566, -24.4562) -> (-176.3566, -37.456)
  spline S160 degree 3 poles (-176.3566, -18.406) (-176.3566, -18.681) (-176.5816, -18.906) (-176.8568, -18.906) knots 0 0 0 0 1 1 1 1
  line L160 (-176.8568, -18.906) -> (-189.8569, -18.906)
  spline S161 degree 3 poles (-189.8569, -18.906) (-190.1318, -18.906) (-190.3568, -18.681) (-190.3568, -18.406) knots 2 2 2 2 3 3 3 3
  line L161 (-190.3568, -18.406) -> (-190.3568, -5.4062)
  spline S162 degree 3 poles (-190.3568, -5.4062) (-190.3568, -5.1311) (-190.1318, -4.9062) (-189.8569, -4.9062) knots 4 4 4 4 5 5 5 5
  line L162 (-189.8569, -4.9062) -> (-176.8568, -4.9062)
  spline S163 degree 3 poles (-176.8568, -4.9062) (-176.5816, -4.9062) (-176.3566, -5.1311) (-176.3566, -5.4062) knots 6 6 6 6 7 7 7 7
  line L163 (-176.3566, -5.4062) -> (-176.3566, -18.406)
  spline S164 degree 3 poles (-176.3566, 24.4559) (-176.3566, 24.1808) (-176.5816, 23.9558) (-176.8568, 23.9558) knots 0 0 0 0 1 1 1 1
  line L164 (-176.8568, 23.9558) -> (-189.8569, 23.9558)
  spline S165 degree 3 poles (-189.8569, 23.9558) (-190.1318, 23.9558) (-190.3568, 24.1808) (-190.3568, 24.4559) knots 2 2 2 2 3 3 3 3
  line L165 (-190.3568, 24.4559) -> (-190.3568, 37.456)
  spline S166 degree 3 poles (-190.3568, 37.456) (-190.3568, 37.7311) (-190.1318, 37.956) (-189.8569, 37.956) knots 4 4 4 4 5 5 5 5
  line L166 (-189.8569, 37.956) -> (-176.8568, 37.956)
  spline S167 degree 3 poles (-176.8568, 37.956) (-176.5816, 37.956) (-176.3566, 37.7311) (-176.3566, 37.456) knots 6 6 6 6 7 7 7 7
  line L167 (-176.3566, 37.456) -> (-176.3566, 24.4559)
  spline S168 degree 3 poles (-9.3813, -24.4562) (-9.3813, -24.1811) (-9.1564, -23.9562) (-8.8815, -23.9562) knots 0 0 0 0 1 1 1 1
  line L168 (-8.8815, -23.9562) -> (4.1183, -23.9562)
  spline S169 degree 3 poles (4.1183, -23.9562) (4.3935, -23.9562) (4.6185, -24.1811) (4.6185, -24.4562) knots 2 2 2 2 3 3 3 3
  line L169 (4.6185, -24.4562) -> (4.6185, -37.456)
  spline S170 degree 3 poles (4.6185, -37.456) (4.6185, -37.7311) (4.3935, -37.956) (4.1183, -37.956) knots 4 4 4 4 5 5 5 5
  line L170 (4.1183, -37.956) -> (-8.8815, -37.956)
  spline S171 degree 3 poles (-8.8815, -37.956) (-9.1564, -37.956) (-9.3813, -37.7311) (-9.3813, -37.456) knots 6 6 6 6 7 7 7 7
  line L171 (-9.3813, -37.456) -> (-9.3813, -24.4562)
  spline S172 degree 3 poles (-14.1445, 32.6938) (-14.1445, 32.9689) (-13.9196, 33.1939) (-13.6447, 33.1939) knots 0 0 0 0 1 1 1 1
  line L172 (-13.6447, 33.1939) -> (-0.6446, 33.1939)
  spline S173 degree 3 poles (-0.6446, 33.1939) (-0.3693, 33.1939) (-0.1443, 32.9689) (-0.1443, 32.6938) knots 2 2 2 2 3 3 3 3
  line L173 (-0.1443, 32.6938) -> (-0.1443, 19.6941)
  spline S174 degree 3 poles (-0.1443, 19.6941) (-0.1443, 19.419) (-0.3693, 19.194) (-0.6446, 19.194) knots 4 4 4 4 5 5 5 5
  line L174 (-0.6446, 19.194) -> (-13.6447, 19.194)
  spline S175 degree 3 poles (-13.6447, 19.194) (-13.9196, 19.194) (-14.1445, 19.419) (-14.1445, 19.6941) knots 6 6 6 6 7 7 7 7
  line L175 (-14.1445, 19.6941) -> (-14.1445, 32.6938)
  spline S176 degree 3 poles (-176.3566, 0.6441) (-176.3566, 0.369) (-176.5816, 0.144) (-176.8568, 0.144) knots 0 0 0 0 1 1 1 1
  line L176 (-176.8568, 0.144) -> (-189.8569, 0.144)
  spline S177 degree 3 poles (-189.8569, 0.144) (-190.1318, 0.144) (-190.3568, 0.369) (-190.3568, 0.6441) knots 2 2 2 2 3 3 3 3
  line L177 (-190.3568, 0.6441) -> (-190.3568, 13.6438)
  spline S178 degree 3 poles (-190.3568, 13.6438) (-190.3568, 13.9189) (-190.1318, 14.1438) (-189.8569, 14.1438) knots 4 4 4 4 5 5 5 5
  line L178 (-189.8569, 14.1438) -> (-176.8568, 14.1438)
  spline S179 degree 3 poles (-176.8568, 14.1438) (-176.5816, 14.1438) (-176.3566, 13.9189) (-176.3566, 13.6438) knots 6 6 6 6 7 7 7 7
  line L179 (-176.3566, 13.6438) -> (-176.3566, 0.6441)
  spline S180 degree 3 poles (-157.3066, -56.506) (-157.3066, -56.7811) (-157.5316, -57.006) (-157.8068, -57.006) knots 0 0 0 0 1 1 1 1
  line L180 (-157.8068, -57.006) -> (-170.8069, -57.006)
  spline S181 degree 3 poles (-170.8069, -57.006) (-171.0818, -57.006) (-171.3068, -56.7811) (-171.3068, -56.506) knots 2 2 2 2 3 3 3 3
  line L181 (-171.3068, -56.506) -> (-171.3068, -43.5062)
  spline S182 degree 3 poles (-171.3068, -43.5062) (-171.3068, -43.2312) (-171.0818, -43.0062) (-170.8069, -43.0062) knots 4 4 4 4 5 5 5 5
  line L182 (-170.8069, -43.0062) -> (-157.8068, -43.0062)
  spline S183 degree 3 poles (-157.8068, -43.0062) (-157.5316, -43.0062) (-157.3066, -43.2312) (-157.3066, -43.5062) knots 6 6 6 6 7 7 7 7
  line L183 (-157.3066, -43.5062) -> (-157.3066, -56.506)
  spline S184 degree 3 poles (62.0555, 56.506) (62.0555, 56.7811) (62.2805, 57.006) (62.5554, 57.006) knots 0 0 0 0 1 1 1 1
  line L184 (62.5554, 57.006) -> (75.5555, 57.006)
  spline S185 degree 3 poles (75.5555, 57.006) (75.8307, 57.006) (76.0557, 56.7811) (76.0557, 56.506) knots 2 2 2 2 3 3 3 3
  line L185 (76.0557, 56.506) -> (76.0557, 43.5059)
  spline S186 degree 3 poles (76.0557, 43.5059) (76.0557, 43.2308) (75.8307, 43.0058) (75.5555, 43.0058) knots 4 4 4 4 5 5 5 5
  line L186 (75.5555, 43.0058) -> (62.5554, 43.0058)
  spline S187 degree 3 poles (62.5554, 43.0058) (62.2805, 43.0058) (62.0555, 43.2308) (62.0555, 43.5059) knots 6 6 6 6 7 7 7 7
  line L187 (62.0555, 43.5059) -> (62.0555, 56.506)
  line L188 (33.4805, 0.6441) -> (33.4805, 13.6438)
  spline S188 degree 3 poles (33.4805, 13.6438) (33.4805, 13.9189) (33.7055, 14.1438) (33.9804, 14.1438) knots 1 1 1 1 2 2 2 2
  line L189 (33.9804, 14.1438) -> (46.9805, 14.1438)
  spline S189 degree 3 poles (46.9805, 14.1438) (47.2557, 14.1438) (47.4807, 13.9189) (47.4807, 13.6438) knots 3 3 3 3 4 4 4 4
  line L190 (47.4807, 13.6438) -> (47.4807, 0.6441)
  spline S190 degree 3 poles (47.4807, 0.6441) (47.4807, 0.369) (47.2557, 0.144) (46.9805, 0.144) knots 5 5 5 5 6 6 6 6
  line L191 (46.9805, 0.144) -> (33.9804, 0.144)
  spline S191 degree 3 poles (33.9804, 0.144) (33.7055, 0.144) (33.4805, 0.369) (33.4805, 0.6441) knots 7 7 7 7 8 8 8 8
  spline S192 degree 3 poles (-33.1946, 56.506) (-33.1946, 56.7811) (-32.9696, 57.006) (-32.6947, 57.006) knots 0 0 0 0 1 1 1 1
  line L192 (-32.6947, 57.006) -> (-19.6946, 57.006)
  spline S193 degree 3 poles (-19.6946, 57.006) (-19.4193, 57.006) (-19.1944, 56.7811) (-19.1944, 56.506) knots 2 2 2 2 3 3 3 3
  line L193 (-19.1944, 56.506) -> (-19.1944, 43.5059)
  spline S194 degree 3 poles (-19.1944, 43.5059) (-19.1944, 43.2308) (-19.4193, 43.0058) (-19.6946, 43.0058) knots 4 4 4 4 5 5 5 5
  line L194 (-19.6946, 43.0058) -> (-32.6947, 43.0058)
  spline S195 degree 3 poles (-32.6947, 43.0058) (-32.9696, 43.0058) (-33.1946, 43.2308) (-33.1946, 43.5059) knots 6 6 6 6 7 7 7 7
  line L195 (-33.1946, 43.5059) -> (-33.1946, 56.506)
  spline S196 degree 3 poles (-174.9321, 43.5059) (-174.9321, 43.2308) (-175.157, 43.0058) (-175.4323, 43.0058) knots 0 0 0 0 1 1 1 1
  line L196 (-175.4323, 43.0058) -> (-190.7823, 43.0058)
  spline S197 degree 3 poles (-190.7823, 43.0058) (-191.0572, 43.0058) (-191.2822, 43.2308) (-191.2822, 43.5059) knots 2 2 2 2 3 3 3 3
  line L197 (-191.2822, 43.5059) -> (-191.2822, 56.506)
  spline S198 degree 3 poles (-191.2822, 56.506) (-191.2822, 56.7811) (-191.0572, 57.006) (-190.7823, 57.006) knots 4 4 4 4 5 5 5 5
  line L198 (-190.7823, 57.006) -> (-175.4323, 57.006)
  spline S199 degree 3 poles (-175.4323, 57.006) (-175.157, 57.006) (-174.9321, 56.7811) (-174.9321, 56.506) knots 6 6 6 6 7 7 7 7
  line L199 (-174.9321, 56.506) -> (-174.9321, 43.5059)
  spline S200 degree 3 poles (-157.3066, -37.456) (-157.3066, -37.7311) (-157.5316, -37.956) (-157.8068, -37.956) knots 0 0 0 0 1 1 1 1
  line L200 (-157.8068, -37.956) -> (-170.8069, -37.956)
  spline S201 degree 3 poles (-170.8069, -37.956) (-171.0818, -37.956) (-171.3068, -37.7311) (-171.3068, -37.456) knots 2 2 2 2 3 3 3 3
  line L201 (-171.3068, -37.456) -> (-171.3068, -24.4562)
  spline S202 degree 3 poles (-171.3068, -24.4562) (-171.3068, -24.1811) (-171.0818, -23.9562) (-170.8069, -23.9562) knots 4 4 4 4 5 5 5 5
  line L202 (-170.8069, -23.9562) -> (-157.8068, -23.9562)
  spline S203 degree 3 poles (-157.8068, -23.9562) (-157.5316, -23.9562) (-157.3066, -24.1811) (-157.3066, -24.4562) knots 6 6 6 6 7 7 7 7
  line L203 (-157.3066, -24.4562) -> (-157.3066, -37.456)
  spline S204 degree 3 poles (-157.3066, -18.406) (-157.3066, -18.681) (-157.5316, -18.906) (-157.8068, -18.906) knots 0 0 0 0 1 1 1 1
  line L204 (-157.8068, -18.906) -> (-170.8069, -18.906)
  spline S205 degree 3 poles (-170.8069, -18.906) (-171.0818, -18.906) (-171.3068, -18.681) (-171.3068, -18.406) knots 2 2 2 2 3 3 3 3
  line L205 (-171.3068, -18.406) -> (-171.3068, -5.4062)
  spline S206 degree 3 poles (-171.3068, -5.4062) (-171.3068, -5.1311) (-171.0818, -4.9062) (-170.8069, -4.9062) knots 4 4 4 4 5 5 5 5
  line L206 (-170.8069, -4.9062) -> (-157.8068, -4.9062)
  spline S207 degree 3 poles (-157.8068, -4.9062) (-157.5316, -4.9062) (-157.3066, -5.1311) (-157.3066, -5.4062) knots 6 6 6 6 7 7 7 7
  line L207 (-157.3066, -5.4062) -> (-157.3066, -18.406)
  spline S208 degree 3 poles (-90.3446, 32.6938) (-90.3446, 32.9689) (-90.1196, 33.1939) (-89.8447, 33.1939) knots 0 0 0 0 1 1 1 1
  line L208 (-89.8447, 33.1939) -> (-76.845, 33.1939)
  spline S209 degree 3 poles (-76.845, 33.1939) (-76.5697, 33.1939) (-76.3447, 32.9689) (-76.3447, 32.6938) knots 2 2 2 2 3 3 3 3
  line L209 (-76.3447, 32.6938) -> (-76.3447, 19.6941)
  spline S210 degree 3 poles (-76.3447, 19.6941) (-76.3447, 19.419) (-76.5697, 19.194) (-76.845, 19.194) knots 4 4 4 4 5 5 5 5
  line L210 (-76.845, 19.194) -> (-89.8447, 19.194)
  spline S211 degree 3 poles (-89.8447, 19.194) (-90.1196, 19.194) (-90.3446, 19.419) (-90.3446, 19.6941) knots 6 6 6 6 7 7 7 7
  line L211 (-90.3446, 19.6941) -> (-90.3446, 32.6938)
  spline S212 degree 3 poles (0.6435, -18.906) (0.3686, -18.906) (0.1437, -18.681) (0.1437, -18.406) knots 0 0 0 0 1 1 1 1
  line L212 (0.1437, -18.406) -> (0.1437, -5.4062)
  spline S213 degree 3 poles (0.1437, -5.4062) (0.1437, -5.1311) (0.3686, -4.9062) (0.6435, -4.9062) knots 2 2 2 2 3 3 3 3
  line L213 (0.6435, -4.9062) -> (13.6433, -4.9062)
  spline S214 degree 3 poles (13.6433, -4.9062) (13.9185, -4.9062) (14.1435, -5.1311) (14.1435, -5.4062) knots 4 4 4 4 5 5 5 5
  line L214 (14.1435, -5.4062) -> (14.1435, -18.406)
  spline S215 degree 3 poles (14.1435, -18.406) (14.1435, -18.681) (13.9185, -18.906) (13.6433, -18.906) knots 6 6 6 6 7 7 7 7
  line L215 (13.6433, -18.906) -> (0.6435, -18.906)
  spline S216 degree 3 poles (23.9555, 56.506) (23.9555, 56.7811) (24.1805, 57.006) (24.4554, 57.006) knots 0 0 0 0 1 1 1 1
  line L216 (24.4554, 57.006) -> (37.4554, 57.006)
  spline S217 degree 3 poles (37.4554, 57.006) (37.7307, 57.006) (37.9557, 56.7811) (37.9557, 56.506) knots 2 2 2 2 3 3 3 3
  line L217 (37.9557, 56.506) -> (37.9557, 43.5059)
  spline S218 degree 3 poles (37.9557, 43.5059) (37.9557, 43.2308) (37.7307, 43.0058) (37.4554, 43.0058) knots 4 4 4 4 5 5 5 5
  line L218 (37.4554, 43.0058) -> (24.4554, 43.0058)
  spline S219 degree 3 poles (24.4554, 43.0058) (24.1805, 43.0058) (23.9555, 43.2308) (23.9555, 43.5059) knots 6 6 6 6 7 7 7 7
  line L219 (23.9555, 43.5059) -> (23.9555, 56.506)
  spline S220 degree 3 poles (-52.2446, 56.506) (-52.2446, 56.7811) (-52.0196, 57.006) (-51.7447, 57.006) knots 0 0 0 0 1 1 1 1
  line L220 (-51.7447, 57.006) -> (-38.7446, 57.006)
  spline S221 degree 3 poles (-38.7446, 57.006) (-38.4693, 57.006) (-38.2444, 56.7811) (-38.2444, 56.506) knots 2 2 2 2 3 3 3 3
  line L221 (-38.2444, 56.506) -> (-38.2444, 43.5059)
  spline S222 degree 3 poles (-38.2444, 43.5059) (-38.2444, 43.2308) (-38.4693, 43.0058) (-38.7446, 43.0058) knots 4 4 4 4 5 5 5 5
  line L222 (-38.7446, 43.0058) -> (-51.7447, 43.0058)
  spline S223 degree 3 poles (-51.7447, 43.0058) (-52.0196, 43.0058) (-52.2446, 43.2308) (-52.2446, 43.5059) knots 6 6 6 6 7 7 7 7
  line L223 (-52.2446, 43.5059) -> (-52.2446, 56.506)
  spline S224 degree 3 poles (19.6936, -18.906) (19.4186, -18.906) (19.1937, -18.681) (19.1937, -18.406) knots 0 0 0 0 1 1 1 1
  line L224 (19.1937, -18.406) -> (19.1937, -5.4062)
  spline S225 degree 3 poles (19.1937, -5.4062) (19.1937, -5.1311) (19.4186, -4.9062) (19.6936, -4.9062) knots 2 2 2 2 3 3 3 3
  line L225 (19.6936, -4.9062) -> (32.6933, -4.9062)
  spline S226 degree 3 poles (32.6933, -4.9062) (32.9686, -4.9062) (33.1935, -5.1311) (33.1935, -5.4062) knots 4 4 4 4 5 5 5 5
  line L226 (33.1935, -5.4062) -> (33.1935, -18.406)
  spline S227 degree 3 poles (33.1935, -18.406) (33.1935, -18.681) (32.9686, -18.906) (32.6933, -18.906) knots 6 6 6 6 7 7 7 7
  line L227 (32.6933, -18.906) -> (19.6936, -18.906)
  spline S228 degree 3 poles (-157.3066, 0.6441) (-157.3066, 0.369) (-157.5316, 0.144) (-157.8068, 0.144) knots 0 0 0 0 1 1 1 1
  line L228 (-157.8068, 0.144) -> (-170.8069, 0.144)
  spline S229 degree 3 poles (-170.8069, 0.144) (-171.0818, 0.144) (-171.3068, 0.369) (-171.3068, 0.6441) knots 2 2 2 2 3 3 3 3
  line L229 (-171.3068, 0.6441) -> (-171.3068, 13.6438)
  spline S230 degree 3 poles (-171.3068, 13.6438) (-171.3068, 13.9189) (-171.0818, 14.1438) (-170.8069, 14.1438) knots 4 4 4 4 5 5 5 5
  line L230 (-170.8069, 14.1438) -> (-157.8068, 14.1438)
  spline S231 degree 3 poles (-157.8068, 14.1438) (-157.5316, 14.1438) (-157.3066, 13.9189) (-157.3066, 13.6438) knots 6 6 6 6 7 7 7 7
  line L231 (-157.3066, 13.6438) -> (-157.3066, 0.6441)
  spline S232 degree 3 poles (100.1555, 32.6938) (100.1555, 32.9689) (100.3805, 33.1939) (100.6554, 33.1939) knots 0 0 0 0 1 1 1 1
  line L232 (100.6554, 33.1939) -> (113.6555, 33.1939)
  spline S233 degree 3 poles (113.6555, 33.1939) (113.9308, 33.1939) (114.1557, 32.9689) (114.1557, 32.6938) knots 2 2 2 2 3 3 3 3
  line L233 (114.1557, 32.6938) -> (114.1557, 19.6941)
  spline S234 degree 3 poles (114.1557, 19.6941) (114.1557, 19.419) (113.9308, 19.194) (113.6555, 19.194) knots 4 4 4 4 5 5 5 5
  line L234 (113.6555, 19.194) -> (100.6554, 19.194)
  spline S235 degree 3 poles (100.6554, 19.194) (100.3805, 19.194) (100.1555, 19.419) (100.1555, 19.6941) knots 6 6 6 6 7 7 7 7
  line L235 (100.1555, 19.6941) -> (100.1555, 32.6938)
  spline S236 degree 3 poles (110.1804, 0.144) (109.9055, 0.144) (109.6805, 0.369) (109.6805, 0.6441) knots 0 0 0 0 1 1 1 1
  line L236 (109.6805, 0.6441) -> (109.6805, 13.6438)
  spline S237 degree 3 poles (109.6805, 13.6438) (109.6805, 13.9189) (109.9055, 14.1438) (110.1804, 14.1438) knots 2 2 2 2 3 3 3 3
  line L237 (110.1804, 14.1438) -> (123.1805, 14.1438)
  spline S238 degree 3 poles (123.1805, 14.1438) (123.4558, 14.1438) (123.6807, 13.9189) (123.6807, 13.6438) knots 4 4 4 4 5 5 5 5
  line L238 (123.6807, 13.6438) -> (123.6807, 0.6441)
  spline S239 degree 3 poles (123.6807, 0.6441) (123.6807, 0.369) (123.4558, 0.144) (123.1805, 0.144) knots 6 6 6 6 7 7 7 7
  line L239 (123.1805, 0.144) -> (110.1804, 0.144)
  spline S240 degree 3 poles (114.4437, -5.4062) (114.4437, -5.1311) (114.6687, -4.9062) (114.9436, -4.9062) knots 0 0 0 0 1 1 1 1
  line L240 (114.9436, -4.9062) -> (127.9434, -4.9062)
  spline S241 degree 3 poles (127.9434, -4.9062) (128.2186, -4.9062) (128.4436, -5.1311) (128.4436, -5.4062) knots 2 2 2 2 3 3 3 3
  line L241 (128.4436, -5.4062) -> (128.4436, -18.406)
  spline S242 degree 3 poles (128.4436, -18.406) (128.4436, -18.681) (128.2186, -18.906) (127.9434, -18.906) knots 4 4 4 4 5 5 5 5
  line L242 (127.9434, -18.906) -> (114.9436, -18.906)
  spline S243 degree 3 poles (114.9436, -18.906) (114.6687, -18.906) (114.4437, -18.681) (114.4437, -18.406) knots 6 6 6 6 7 7 7 7
  line L243 (114.4437, -18.406) -> (114.4437, -5.4062)
  spline S244 degree 3 poles (100.1555, 56.506) (100.1555, 56.7811) (100.3805, 57.006) (100.6554, 57.006) knots 0 0 0 0 1 1 1 1
  line L244 (100.6554, 57.006) -> (113.6555, 57.006)
  spline S245 degree 3 poles (113.6555, 57.006) (113.9308, 57.006) (114.1557, 56.7811) (114.1557, 56.506) knots 2 2 2 2 3 3 3 3
  line L245 (114.1557, 56.506) -> (114.1557, 43.5059)
  spline S246 degree 3 poles (114.1557, 43.5059) (114.1557, 43.2308) (113.9308, 43.0058) (113.6555, 43.0058) knots 4 4 4 4 5 5 5 5
  line L246 (113.6555, 43.0058) -> (100.6554, 43.0058)
  spline S247 degree 3 poles (100.6554, 43.0058) (100.3805, 43.0058) (100.1555, 43.2308) (100.1555, 43.5059) knots 6 6 6 6 7 7 7 7
  line L247 (100.1555, 43.5059) -> (100.1555, 56.506)
  spline S248 degree 3 poles (4.9055, 56.506) (4.9055, 56.7811) (5.1304, 57.006) (5.4054, 57.006) knots 0 0 0 0 1 1 1 1
  line L248 (5.4054, 57.006) -> (18.4054, 57.006)
  spline S249 degree 3 poles (18.4054, 57.006) (18.6807, 57.006) (18.9057, 56.7811) (18.9057, 56.506) knots 2 2 2 2 3 3 3 3
  line L249 (18.9057, 56.506) -> (18.9057, 43.5059)
  spline S250 degree 3 poles (18.9057, 43.5059) (18.9057, 43.2308) (18.6807, 43.0058) (18.4054, 43.0058) knots 4 4 4 4 5 5 5 5
  line L250 (18.4054, 43.0058) -> (5.4054, 43.0058)
  spline S251 degree 3 poles (5.4054, 43.0058) (5.1304, 43.0058) (4.9055, 43.2308) (4.9055, 43.5059) knots 6 6 6 6 7 7 7 7
  line L251 (4.9055, 43.5059) -> (4.9055, 56.506)
  spline S252 degree 3 poles (-42.2197, 0.144) (-42.4946, 0.144) (-42.7196, 0.369) (-42.7196, 0.6441) knots 0 0 0 0 1 1 1 1
  line L252 (-42.7196, 0.6441) -> (-42.7196, 13.6438)
  spline S253 degree 3 poles (-42.7196, 13.6438) (-42.7196, 13.9189) (-42.4946, 14.1438) (-42.2197, 14.1438) knots 2 2 2 2 3 3 3 3
  line L253 (-42.2197, 14.1438) -> (-29.2196, 14.1438)
  spline S254 degree 3 poles (-29.2196, 14.1438) (-28.9443, 14.1438) (-28.7194, 13.9189) (-28.7194, 13.6438) knots 4 4 4 4 5 5 5 5
  line L254 (-28.7194, 13.6438) -> (-28.7194, 0.6441)
  spline S255 degree 3 poles (-28.7194, 0.6441) (-28.7194, 0.369) (-28.9443, 0.144) (-29.2196, 0.144) knots 6 6 6 6 7 7 7 7
  line L255 (-29.2196, 0.144) -> (-42.2197, 0.144)
  spline S256 degree 3 poles (43.0055, 32.6938) (43.0055, 32.9689) (43.2305, 33.1939) (43.5054, 33.1939) knots 0 0 0 0 1 1 1 1
  line L256 (43.5054, 33.1939) -> (56.5055, 33.1939)
  spline S257 degree 3 poles (56.5055, 33.1939) (56.7807, 33.1939) (57.0057, 32.9689) (57.0057, 32.6938) knots 2 2 2 2 3 3 3 3
  line L257 (57.0057, 32.6938) -> (57.0057, 19.6941)
  spline S258 degree 3 poles (57.0057, 19.6941) (57.0057, 19.419) (56.7807, 19.194) (56.5055, 19.194) knots 4 4 4 4 5 5 5 5
  line L258 (56.5055, 19.194) -> (43.5054, 19.194)
  spline S259 degree 3 poles (43.5054, 19.194) (43.2305, 19.194) (43.0055, 19.419) (43.0055, 19.6941) knots 6 6 6 6 7 7 7 7
  line L259 (43.0055, 19.6941) -> (43.0055, 32.6938)
  spline S260 degree 3 poles (-37.9564, -5.4062) (-37.9564, -5.1311) (-37.7314, -4.9062) (-37.4565, -4.9062) knots 0 0 0 0 1 1 1 1
  line L260 (-37.4565, -4.9062) -> (-24.4567, -4.9062)
  spline S261 degree 3 poles (-24.4567, -4.9062) (-24.1815, -4.9062) (-23.9565, -5.1311) (-23.9565, -5.4062) knots 2 2 2 2 3 3 3 3
  line L261 (-23.9565, -5.4062) -> (-23.9565, -18.406)
  spline S262 degree 3 poles (-23.9565, -18.406) (-23.9565, -18.681) (-24.1815, -18.906) (-24.4567, -18.906) knots 4 4 4 4 5 5 5 5
  line L262 (-24.4567, -18.906) -> (-37.4565, -18.906)
  spline S263 degree 3 poles (-37.4565, -18.906) (-37.7314, -18.906) (-37.9564, -18.681) (-37.9564, -18.406) knots 6 6 6 6 7 7 7 7
  line L263 (-37.9564, -18.406) -> (-37.9564, -5.4062)
  spline S264 degree 3 poles (-33.1946, 32.6938) (-33.1946, 32.9689) (-32.9696, 33.1939) (-32.6947, 33.1939) knots 0 0 0 0 1 1 1 1
  line L264 (-32.6947, 33.1939) -> (-19.6946, 33.1939)
  spline S265 degree 3 poles (-19.6946, 33.1939) (-19.4193, 33.1939) (-19.1944, 32.9689) (-19.1944, 32.6938) knots 2 2 2 2 3 3 3 3
  line L265 (-19.1944, 32.6938) -> (-19.1944, 19.6941)
  spline S266 degree 3 poles (-19.1944, 19.6941) (-19.1944, 19.419) (-19.4193, 19.194) (-19.6946, 19.194) knots 4 4 4 4 5 5 5 5
  line L266 (-19.6946, 19.194) -> (-32.6947, 19.194)
  spline S267 degree 3 poles (-32.6947, 19.194) (-32.9696, 19.194) (-33.1946, 19.419) (-33.1946, 19.6941) knots 6 6 6 6 7 7 7 7
  line L267 (-33.1946, 19.6941) -> (-33.1946, 32.6938)